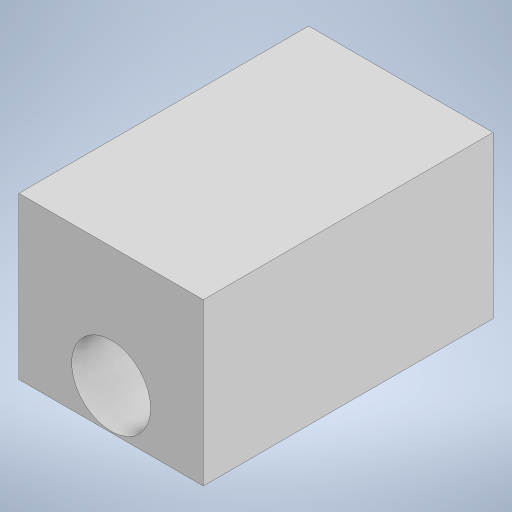
# Autodesk Inventor part: uchwyt silnikow
Saved by Autodesk Inventor 2023 (Build 270158000, 158)
## iProperties
Created: 2023-07-31
Part Number: uchwyt silnikow
Material: Ogólny
Document SubType Name: Modeling
Designer: Kamil
Density: 1 g/cm^3
Appearance: Domyślna
Author: Kamil
Autodesk Inventor part; units mm, degrees
ref_plane "YZ Plane" through (0, 0, 0) normal (1, 0, 0) x (0, 1, 0)
ref_plane "XZ Plane" through (0, 0, 0) normal (0, 1, 0) x (-1, 0, 0)
ref_plane "XY Plane" through (0, 0, 0) normal (0, 0, 1) x (1, 0, 0)
sketch "Szkic1" plane through (0, 0, 0) normal (0, 1, 0) x (-1, 0, 0)
  line L0 (0, 0) -> (-14, 0)
  line L1 (-14, 0) -> (-14, 22)
  line L2 (-14, 22) -> (0, 22)
  line L3 (0, 22) -> (0, 0)
  dimension "d0" = 14
  dimension "d1" = 22
  constraints: 8 end point, 2 parallel, 1 horizontal, 1 perpendicular
  measures "d0" distance of L1.end L2.end
  measures "d1" distance of L2.end L0.start
extrude "Wyciągnięcie proste1" add sketch "Szkic1" along normal blind 8.25
sketch "Szkic2" plane through (0, 0, 22) normal (0, 0, 1) x (1, 0, 0)
  circle A0 centre (7, 3.1) radius 1 projected
  arc A1 (8, 0.2716) -> (6, 0.2716) centre (7, 3.1) ccw projected
  line L0 (6, 0.2716) -> (6, 0) projected
  line L1 (6, 0) -> (8, 0) projected
  line L2 (8, 0) -> (8, 0.2716) projected
  circle A2 centre (7, 3.1) radius 3
  point P0 (0, 0)
  point P1 (6, 0.2716)
  constraints: 1 coincident, 3 other
extrude "Wyciągnięcie proste2" cut sketch "Szkic2" against normal through all contours A0 | A2 A1
sketch "Szkic3" plane through (0, 8.25, 0) normal (0, 1, 0) x (1, 0, 0)
  line L0 (0, -22) -> (14, -22) projected
  line L1 (14, -22) -> (14, 0) projected
  line L2 (14, 0) -> (0, 0) projected
  line L3 (0, 0) -> (0, -22) projected
extrude "Wyciągnięcie proste3" add sketch "Szkic3" along normal blind 4
